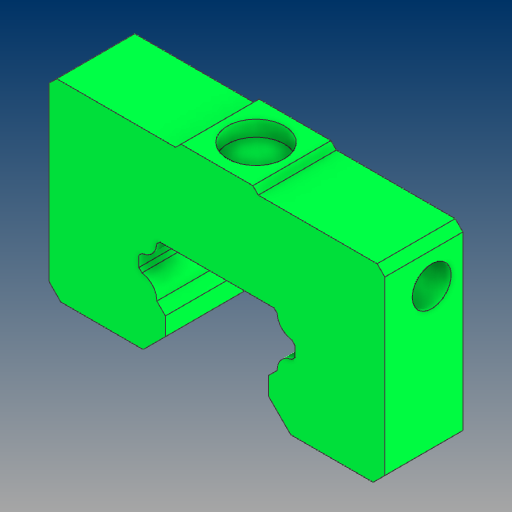
# Autodesk Inventor part: HGR20B
Saved by Autodesk Inventor 2021 (Build 250183000, 183)
## iProperties
Created: 2021-09-26
Part Number: HGR20B
Material: Generic
Document SubType Name: Modeling
Designer: 41601100
Density: 1 g/cm^3
Appearance: Default
Author: 41601100
Autodesk Inventor part; units mm, degrees
ref_plane "YZ Plane" through (0, 0, 0) normal (1, 0, 0) x (0, 1, 0)
ref_plane "XZ Plane" through (0, 0, 0) normal (0, 1, 0) x (-1, 0, 0)
ref_plane "XY Plane" through (0, 0, 0) normal (0, 0, 1) x (1, 0, 0)
sketch "Sketch1" plane through (0, 0, 0) normal (0, 0, 1) x (1, 0, 0)
  line L0 (-5.3, 15) -> (-20.5165, 15)
  line L1 (-4.6, 15.7) -> (-5.3, 15)
  line L2 (4.6, 15.7) -> (-4.6, 15.7)
  line L3 (5.3, 15) -> (4.6, 15.7)
  line L4 (20.5165, 15) -> (5.3, 15)
  line L5 (21.5, 14.0165) -> (20.5165, 15)
  line L6 (21.5, -8) -> (21.5, 14.0165)
  line L7 (20, -9.5) -> (21.5, -8)
  line L8 (9.45, -9.5) -> (20, -9.5)
  line L9 (6.6, -6.65) -> (9.45, -9.5)
  line L10 (6.6, -4.35) -> (6.6, -6.65)
  line L11 (7.7, -3.25) -> (6.6, -4.35)
  arc A0 (9.6, -1.075) -> (7.7, -3.25) centre (9.8292, -3.1926) ccw
  line L12 (10, -0.675) -> (9.6, -1.075)
  line L13 (10, 0.675) -> (10, -0.675)
  line L14 (9.6, 1.075) -> (10, 0.675)
  arc A1 (7.7, 3.1) -> (9.6, 1.075) centre (9.828, 3.1928) ccw
  line L15 (7.3, 3.5) -> (7.7, 3.1)
  line L16 (-7.3, 3.5) -> (7.3, 3.5)
  line L17 (-7.7, 3.1) -> (-7.3, 3.5)
  arc A2 (-9.6, 1.075) -> (-7.7, 3.1) centre (-9.828, 3.1928) ccw
  line L18 (-10, 0.675) -> (-9.6, 1.075)
  line L19 (-10, -0.675) -> (-10, 0.675)
  line L20 (-9.6, -1.075) -> (-10, -0.675)
  arc A3 (-7.7, -3.25) -> (-9.6, -1.075) centre (-9.8292, -3.1926) ccw
  line L21 (-6.6, -4.35) -> (-7.7, -3.25)
  line L22 (-6.6, -6.65) -> (-6.6, -4.35)
  line L23 (-9.45, -9.5) -> (-6.6, -6.65)
  line L24 (-20, -9.5) -> (-9.45, -9.5)
  line L25 (-21.5, -8) -> (-20, -9.5)
  line L26 (-21.5, 14.0165) -> (-21.5, -8)
  line L27 (-20.5165, 15) -> (-21.5, 14.0165)
  point P0 (0, 0)
  point P1 (0, 0)
  constraints: 56 end point, 8 point on circle, 4 centre point
extrude "Extrusion1" add sketch "Sketch1" along normal blind 10
sketch "Sketch2" plane through (-21.5, -8, 0) normal (-1, 0, 0) x (0, 0, 1)
  line L0 (0, 22.0165) -> (0, 0) projected
  line L1 (0, 0) -> (10, 0) projected
  line L2 (10, 22.0165) -> (10, 0) projected
  line L3 (0, 22.0165) -> (10, 22.0165) projected
  line L4 (10, 0) -> (10, 22.0165)
  line L5 (0, 22.0165) -> (10, 22.0165)
  line L6 (0, 0) -> (0, 22.0165)
  line L7 (0, 0) -> (10, 0)
  circle A0 centre (4, 18) radius 2.5
  point P0 (0, 8)
  constraints: 8 end point, 1 centre point
extrude "Extrusion2" cut sketch "Sketch2" against normal blind 6.7 contours A0
mirror "Mirror1" about plane through (0, 0, 0) normal (1, 0, 0) of "Extrusion2"
sketch "Sketch3" plane through (-4.6, 15.7, 0) normal (0, 1, 0) x (1, 0, 0)
  line L0 (9.2, 0) -> (0, 0) projected
  line L1 (0, 0) -> (0, -10) projected
  line L2 (9.2, -10) -> (0, -10) projected
  line L3 (9.2, 0) -> (9.2, -10) projected
  line L4 (0, -10) -> (9.2, -10)
  line L5 (9.2, 0) -> (9.2, -10)
  line L6 (0, 0) -> (9.2, 0)
  line L7 (0, 0) -> (0, -10)
  circle A0 centre (4.6, -5) radius 3.65
  point P0 (4.6, 0)
  constraints: 8 end point, 1 centre point
extrude "Extrusion3" cut sketch "Sketch3" against normal blind 2 contours A0
body "Solid1"
